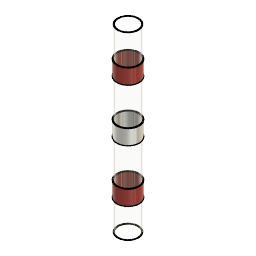
FA7 - 22-16 Gauge Heat Shrink Solder Seal (Autodesk Fusion 360 design; units mm, degrees)
Autodesk Fusion 360 part; units mm, degrees
sketch "Sketch1" plane through (0, 0, 0) normal (0, 0, 1) x (1, 0, 0)
  circle A0 centre (0, 0) radius 0.6455
  circle A1 centre (0, 0) radius 0.7
  dimension "d1" = 1.291
  dimension "d2" = 1.4
  constraint coincident A0.centre A1.centre
  measures "d1" diameter of A0
  measures "d2" diameter of A1
extrude "Extrude1" add sketch "Sketch1" along normal blind 12 makes body 1
sketch "Sketch2" plane through (0, 0, 0) normal (0, 0, 1) x (1, 0, 0)
  circle A0 centre (0, 0) radius 0.7
  circle A1 centre (0, 0) radius 0.75
  dimension "d5" = 1.4
  dimension "d6" = 1.5
  constraint coincident A0.centre A1.centre
  measures "d5" diameter of A0
  measures "d6" diameter of A1
extrude "Extrude2" add sketch "Sketch2" along normal blind 1 from surface at 2 separate body makes body 2
extrude "Extrude3" add sketch "Sketch2" against normal blind 1 from surface at 10 separate body makes body 3
extrude "Extrude4" add sketch "Sketch2" along normal mid plane 1 from surface at 6 separate body makes body 4
